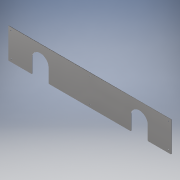
# Autodesk Inventor part: Cover_LeftRight
Saved by Autodesk Inventor 2018 (Build 220112000, 112)
## iProperties
Created: 2017-11-14
Part Number: Cover_LeftRight
Material: Steel, Galvanized
Document SubType Name: Modeling
Designer: P136265
Density: 7.85 g/cm^3
Appearance: Galvanized
Author: P136265
Autodesk Inventor part; units mm, degrees
ref_plane "YZ Plane" through (0, 0, 0) normal (1, 0, 0) x (0, 1, 0)
ref_plane "XZ Plane" through (0, 0, 0) normal (0, 1, 0) x (-1, 0, 0)
ref_plane "XY Plane" through (0, 0, 0) normal (0, 0, 1) x (1, 0, 0)
sketch "Sketch1" plane through (0, 0, 0) normal (0, 1, 0) x (-1, 0, 0)
  line L0 (-414.3, 17.5) -> (-414.3, 107.5) construction
  line L1 (-417.5, -14.3) -> (417.5, -14.3) construction
  line L2 (417.5, 139.3) -> (-417.5, 139.3) construction
  line L3 (414.3, 107.5) -> (414.3, 17.5) construction
  line L4 (417.5, 110.7) -> (-417.5, 110.7) construction
  circle A0 centre (-400, 0) radius 2 construction
  circle A1 centre (-400, 125) radius 2 construction
  circle A2 centre (400, 0) radius 2 construction
  circle A3 centre (400, 125) radius 2 construction
  circle A4 centre (0, 125) radius 2 construction
  circle A5 centre (0, 0) radius 2 construction
  arc A6 (-255.8176, 91.7662) -> (-287.0162, 60.5676) centre (-251.75, 56.5) ccw construction
  arc A7 (-247.75, 95.5) -> (-255.75, 95.5) centre (-251.75, 95.5) ccw construction
  arc A8 (255.75, 95.5) -> (247.75, 95.5) centre (251.75, 95.5) ccw construction
  line L5 (417.5, 14.3) -> (-417.5, 14.3) construction
  line L6 (0, -14.3) -> (0, 139.3) construction
  line L7 (-414.3, 139.3) -> (414.3, 139.3)
  line L8 (414.3, 139.3) -> (414.3, -14.3)
  line L9 (-414.3, -14.3) -> (-414.3, 139.3)
  line L10 (-414.3, 139.3) -> (414.3, -14.3) construction
  line L11 (414.3, 139.3) -> (-414.3, -14.3) construction
  line L12 (-251.75, 99.5) -> (-251.75, 14.3) construction
  line L13 (251.75, 99.5) -> (251.75, 14.3) construction
  line L14 (-294.75, 56.5) -> (-294.75, -14.3)
  line L15 (-208.75, 56.5) -> (-208.75, -14.3)
  line L16 (209.15, 56.9) -> (209.15, -14.3)
  line L17 (294.35, 56.9) -> (294.35, -14.3)
  arc A9 (-260.011, 14.301) -> (-260.0059, 14.3) centre (-251.75, 56.5) ccw
  arc A10 (-208.75, 56.5) -> (-294.75, 56.5) centre (-251.75, 56.5) ccw
  arc A11 (294.35, 56.9) -> (209.15, 56.9) centre (251.75, 56.9) ccw
  line L18 (-294.75, -14.3) -> (-414.3, -14.3)
  line L19 (414.3, -14.3) -> (294.35, -14.3)
  line L20 (209.15, -14.3) -> (-208.75, -14.3)
  circle A12 centre (-400, 0) radius 3
  circle A13 centre (-400, 125) radius 3
  circle A14 centre (0, 0) radius 3
  circle A15 centre (0, 125) radius 3
  circle A16 centre (400, 125) radius 3
  circle A17 centre (400, 0) radius 3
  point P0 (0, 0)
  point P1 (0, 62.5)
  dimension "d0" = 828.6
  dimension "d1" = 43
  dimension "d2" = 125
  dimension "d3" = 1
  dimension "d4" = 1
  dimension "d5" = 1
  dimension "d6" = 1
  dimension "d7" = 1
  dimension "d8" = 1
  constraints: 30 end point, 10 point on circle, 9 centre point, 9 perpendicular, 6 midpoint, 6 point on line, 4 parallel, 4 tangent, 1 coincident, 1 horizontal
  measures "d0" distance of L7.start L7.end
  measures "d1" radius of A9
  measures "d2" distance between parallel lines of L4 L20
  measures "d3" radial gap between concentric circles of A0 A12
  measures "d4" radial gap between concentric circles of A1 A13
  measures "d5" radial gap between concentric circles of A5 A14
  measures "d6" radial gap between concentric circles of A4 A15
  measures "d7" radial gap between concentric circles of A3 A16
  measures "d8" radial gap between concentric circles of A2 A17
extrude "Extrusion1" add sketch "Sketch1" along normal mid plane 2
fillet "Fillet1" radius 2 8 edges at (414.3, 0, -14.3) (208.75, 0, -14.3) (294.75, 0, -14.3) (-209.15, 0, -14.3) (-294.35, 0, -14.3) (-414.3, 0, -14.3) (414.3, 0, 139.3) (-414.3, 0, 139.3)
body "Solid1"
